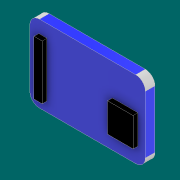
# Autodesk Inventor part: AmplificadorFInal
Saved by Autodesk Inventor 2020 (Build 240168000, 168)
## iProperties
Created: 2021-02-09
Part Number: AmplificadorFInal
Material: Generic
Document SubType Name: Modeling
Designer: santi
Density: 1 g/cm^3
Appearance: Default
Author: santi
Autodesk Inventor part; units mm, degrees
ref_plane "YZ Plane" through (0, 0, 0) normal (1, 0, 0) x (0, 1, 0)
ref_plane "XZ Plane" through (0, 0, 0) normal (0, 1, 0) x (-1, 0, 0)
ref_plane "XY Plane" through (0, 0, 0) normal (0, 0, 1) x (1, 0, 0)
sketch "Sketch1" plane through (0, 0, 0) normal (0, 0, 1) x (1, 0, 0)
  line L0 (0, 0) -> (24, 0)
  line L1 (24, 0) -> (24, 16)
  line L2 (24, 16) -> (0, 16)
  line L3 (0, 16) -> (0, 0)
  dimension "d0" = 24
  dimension "d1" = 16
  constraints: 8 end point, 3 perpendicular, 1 horizontal
  measures "d0" distance of L0.start L0.end
  measures "d1" distance of L0.end L1.end
extrude "Extrusion1" add sketch "Sketch1" along normal blind 2
fillet "Fillet1" radius 2 4 edges at (0, 16, 1) (0, 0, 1) (24, 0, 1) (24, 16, 1)
sketch "Sketch2" plane through (0, 0, 2) normal (0, 0, 1) x (1, 0, 0)
  line L0 (1.8518, 13.3448) -> (1.8518, 2.0387)
  line L1 (1.8518, 2.0387) -> (3.5541, 2.0387)
  line L2 (3.5541, 2.0387) -> (3.5541, 13.3448)
  line L3 (3.5541, 13.3448) -> (1.8518, 13.3448)
  line L4 (17.1468, 9.3813) -> (17.1468, 3.3599)
  line L5 (17.1468, 3.3599) -> (22.4569, 3.3599)
  line L6 (22.4569, 3.3599) -> (22.4569, 9.3813)
  line L7 (22.4569, 9.3813) -> (17.1468, 9.3813)
  point P0 (0, 0)
  constraints: 16 end point, 6 perpendicular, 2 vertical
extrude "Extrusion2" add sketch "Sketch2" along normal blind 1
body "Solid1"
